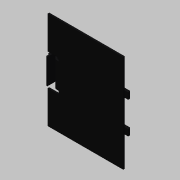
# Autodesk Inventor part: BAcA_3
Saved by Autodesk Inventor 2019.3 (Build 233278000, 278)
## iProperties
Created: 2019-02-21
Part Number: BAcA_3
Material: Generic
Document SubType Name: Modeling
Designer: Varga Daniel
Density: 1 g/cm^3
Appearance: Default
Author: Varga Daniel
Autodesk Inventor part; units mm, degrees
ref_plane "YZ Plane" through (0, 0, 0) normal (1, 0, 0) x (0, 1, 0)
ref_plane "XZ Plane" through (0, 0, 0) normal (0, 1, 0) x (-1, 0, 0)
ref_plane "XY Plane" through (0, 0, 0) normal (0, 0, 1) x (1, 0, 0)
ref_plane "Work Plane1" through (0, 0, 0) normal (0, 0, 1) x (1, 0, 0)
sketch "Sketch1" plane through (0, 0, 0) normal (0, 0, 1) x (1, 0, 0)
  line L0 (-60, -72.111) -> (-60, -152.111) construction
  line L1 (0, -152.111) -> (-60, -152.111) construction
  line L2 (0, -72.111) -> (0, -152.111) construction
  line L3 (-57, -81.311) -> (-9.2, -81.311)
  line L4 (-9.2, -81.311) -> (-9.2, -142.911)
  line L5 (-9.2, -142.911) -> (-57, -142.911)
  line L6 (-57, -142.911) -> (-57, -81.311)
  line L7 (-57, -112.111) -> (-9.2, -112.111) construction
  line L8 (-57, -102.111) -> (-50, -102.111)
  line L9 (-50, -102.111) -> (-50, -122.111)
  line L10 (-50, -122.111) -> (-57, -122.111)
  line L11 (-57, -122.111) -> (-57, -102.111)
  line L12 (0, -72.111) -> (-60, -72.111) projected
  line L13 (-9.2, -81.311) -> (-57, -81.311) projected
  line L14 (-9.2, -142.911) -> (-9.2, -81.311) projected
  line L15 (-57, -142.911) -> (-9.2, -142.911) projected
  line L16 (-57, -81.311) -> (-57, -142.911) projected
  point P0 (0, 0)
  dimension "d0" = 20
  dimension "d1" = 7
  constraints: 18 end point, 4 parallel, 2 horizontal, 2 midpoint, 2 perpendicular, 1 point on line, 2 other
  measures "d0" distance between parallel lines of L10 L8
  measures "d1" distance between parallel lines of L11 L9
extrude "Extrusion1" add sketch "Sketch1" against normal blind 1 contours L3 L4 L5 L6 L10 L9 L8
ref_plane "Work Plane2" through (-57, -112.111, 0) normal (0, 1, 0) x (1, 0, 0)
sketch "Sketch2" plane through (-57, -112.111, 0) normal (0, 1, 0) x (1, 0, 0)
  line L0 (7, 0) -> (0, 0) construction
  line L1 (7, 0) -> (7, 1) construction
  line L2 (0, 1) -> (7, 1) construction
  line L3 (0, 0) -> (0, 1) construction
  line L4 (0.0721, -0.8167) -> (0.0721, 1.0988)
  line L5 (0.0721, 1.0988) -> (-0.9279, 1.3644)
  line L6 (-0.9279, 1.3644) -> (0.0477, 5.0375)
  arc A0 (1.8249, 5.3661) -> (0.0477, 5.0375) centre (1.0142, 4.7807) ccw
  line L7 (1.8249, 5.3661) -> (4.3785, 1.8293)
  arc A1 (4.3785, 1.8293) -> (6, 1) centre (6, 3) ccw
  line L8 (6, 1) -> (7, 1)
  line L9 (7, 1) -> (7, 0)
  line L10 (7, 0) -> (6, 0)
  arc A2 (3.5677, 1.2439) -> (6, 0) centre (6, 3) ccw
  line L11 (3.5677, 1.2439) -> (1.0644, 4.7112)
  arc A3 (1.0644, 4.7112) -> (0.9749, 4.6822) centre (1.0243, 4.6822) ccw
  line L12 (47.8, 0) -> (0, 0) projected
  line L13 (47.8, 1) -> (0, 1) projected
  line L14 (6, 0) -> (6, 1) construction
  line L15 (0.9749, -0.9502) -> (0.9749, 4.6822)
  line L16 (0.2208, -1.01) -> (0.7236, -1.1435)
  arc A4 (0.7236, -1.1435) -> (0.9749, -0.9502) centre (0.7749, -0.9502) ccw
  arc A5 (0.0721, -0.8167) -> (0.2208, -1.01) centre (0.2721, -0.8167) ccw
  point P0 (57, 0)
  point P1 (0.9749, -1.2103)
  point P2 (0.0721, -0.9705)
  dimension "d8" = 1
  dimension "d9" = 1
  dimension "d11" = 1
  dimension "d12" = 0.0494
  dimension "d22" = 1
  dimension "d23" = 2
  dimension "d32" = 2
  dimension "d34" = 2.5
  dimension "d36" = 0.2
  dimension "d37" = 0.9874
  dimension "d38" = 1
  dimension "d39" = 125.829
  dimension "d40" = 3.8003
  constraints: 20 end point, 12 point on circle, 12 tangent, 6 centre point, 4 parallel, 4 point on line, 2 collinear, 2 horizontal, 1 equal radius, 6 other
  measures "d8" distance between parallel lines of L11 L7
  measures "d9" distance between parallel lines of L8 L10
  measures "d11" radius of A0
  measures "d12" radius of A3
  measures "d22" distance from line of L4 L6.start
  measures "d23" radius of A1
  measures "d34" distance from line of point (0.975, -1.21) L6
  measures "d36" radius of A4
  measures "d37" distance from line of L15.end L6
  measures "d38" distance between parallel lines of L1 L14
  measures "d39" angle to the sketch x axis of L7
extrude "Extrusion2" add sketch "Sketch2" along normal mid plane 16 contours L4 L12 L15 A4 L16 A5 | L4 L13 L15 L12 | L4 L5 L6 A0 L7 A1 L13 A2 L11 A3 L15 | A2 L13 L8 L9 L10
ref_plane "Work Plane3" through (-57, -102.111, 0) normal (0, 1, 0) x (1, 0, 0)
sketch "Sketch4" plane through (-57, -102.111, 0) normal (0, 1, 0) x (1, 0, 0)
  line L0 (57, 0) -> (-3, 0) construction
  line L1 (0, 0) -> (47.8, 0) construction
  line L2 (47.8, 0) -> (47.8, 1) construction
  line L3 (0, 1) -> (47.8, 1) construction
  line L4 (0, 0) -> (0, 1) construction
  line L5 (0, 1) -> (47.8, 1) projected
  line L6 (45.8, 1) -> (47.8, 1)
  line L7 (47.8, 1) -> (49.8, 1)
  line L8 (49.8, 1) -> (49.8, 2.1)
  line L9 (49.4, 2.5) -> (46.2, 2.5)
  line L10 (45.8, 2.1) -> (45.8, 1)
  arc A0 (49.8, 2.1) -> (49.4, 2.5) centre (49.4, 2.1) ccw
  arc A1 (46.2, 2.5) -> (45.8, 2.1) centre (46.2, 2.1) ccw
  point P0 (49.8, 2.5)
  dimension "d25" = 1.5
  dimension "d26" = 2
  dimension "d27" = 2
  dimension "d28" = 0.4
  constraints: 10 end point, 4 point on circle, 4 point on line, 4 tangent, 3 perpendicular, 2 centre point, 1 collinear, 1 equal radius
  measures "d25" distance of L7.end point (49.8, 2.5)
  measures "d26" distance between parallel lines of L2 L8
  measures "d27" distance between parallel lines of L2 L10
  measures "d28" radius of A0
extrude "Extrusion3" add sketch "Sketch4" along normal mid plane 4
mirror "Mirror1" about plane through (-57, -112.111, 0) normal (0, 1, 0) of "Extrusion3"
thicken "Thicken1" operation add thickness 0.1 both sides no extend neighbours yes toward (0, 1, 0) faces at (-25.1333, -142.911, -0.3333) (-57, -135.9777, -0.3333) (-9.2, -108.111, -0.3333) (-41.0667, -81.311, -0.3333) (-57, -95.1777, -0.3333)
equation "\"d8\" = d9"
body "Solid1"
